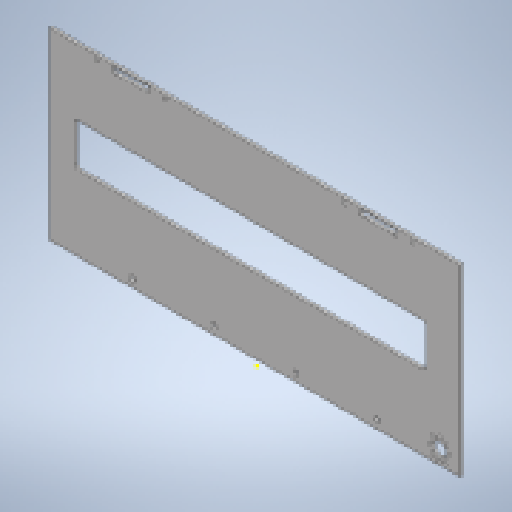
# Autodesk Inventor part: wall2
Saved by Autodesk Inventor 2024 (Build 280153000, 153)
## iProperties
Created: 2024-06-08
Part Number: wall2
Material: 一般
Document SubType Name: モデリング
Designer: right
Density: 1 g/cm^3
Appearance: 既定
Author: right
Autodesk Inventor part; units mm, degrees
ref_plane "YZ Plane" through (0, 0, 0) normal (1, 0, 0) x (0, 1, 0)
ref_plane "XZ Plane" through (0, 0, 0) normal (0, 1, 0) x (-1, 0, 0)
ref_plane "XY Plane" through (0, 0, 0) normal (0, 0, 1) x (1, 0, 0)
sketch "スケッチ1" plane through (0, 0, 0) normal (0, 0, 1) x (1, 0, 0)
  circle A0 centre (71.625, 9) radius 1.3 projected
  circle A1 centre (23.875, 9) radius 1.3 projected
  circle A2 centre (-23.875, 9) radius 1.3 projected
  circle A3 centre (-71.625, 9) radius 1.3 projected
  circle A4 centre (52.5, 109.3641) radius 0.7835 projected
  circle A5 centre (92.5, 109.3641) radius 0.7835 projected
  line L0 (62.5, 107.8641) -> (82.5, 107.8641) projected
  line L1 (82.5, 110.8641) -> (82.5, 107.8641) projected
  line L2 (62.5, 110.8641) -> (82.5, 110.8641) projected
  line L3 (62.5, 110.8641) -> (62.5, 107.8641) projected
  line L4 (-82.5, 107.8641) -> (-62.5, 107.8641) projected
  line L5 (-62.5, 110.8641) -> (-62.5, 107.8641) projected
  line L6 (-82.5, 110.8641) -> (-62.5, 110.8641) projected
  line L7 (-82.5, 110.8641) -> (-82.5, 107.8641) projected
  circle A6 centre (-92.5, 109.3641) radius 0.7835 projected
  circle A7 centre (-52.5, 109.3641) radius 0.7835 projected
  circle A8 centre (64.0053, 60.7224) radius 10 projected
  arc A9 (100, 57.7224) -> (100, 63.7224) centre (100, 60.7224) ccw projected
  circle A10 centre (100, 60.7224) radius 12.5
  arc A11 (-100, 63.7224) -> (-100, 57.7224) centre (-100, 60.7224) ccw projected
  circle A12 centre (-100, 60.7224) radius 12.5
  line L8 (100, 48.2224) -> (-100, 48.2224)
  line L9 (100, 73.2224) -> (-100, 73.2224)
  circle A13 centre (71.625, 9) radius 1.6
  circle A14 centre (23.875, 9) radius 1.6
  circle A15 centre (-23.875, 9) radius 1.6
  circle A16 centre (-71.625, 9) radius 1.6
  circle A17 centre (-92.5, 109.3641) radius 1.1
  circle A18 centre (-52.5, 109.3641) radius 1.1
  circle A19 centre (52.5, 109.3641) radius 1.1
  circle A20 centre (92.5, 109.3641) radius 1.1
  circle A21 centre (82.1, 110.4641) radius 1.1
  line L10 (82.5, 109.3641) -> (62.5, 109.3641) construction
  line L11 (82.1, 110.4641) -> (82.5, 110.8641) construction
  circle A22 centre (82.1, 108.2641) radius 1.1
  line L12 (72.5, 107.8641) -> (72.5, 109.3641) construction
  circle A23 centre (62.9, 110.4641) radius 1.1
  line L13 (62.5, 109.3641) -> (82.5, 109.3641) construction
  circle A24 centre (62.9, 108.2641) radius 1.1
  line L14 (-60.3, 107.8641) -> (60.3, 107.8641) construction
  line L15 (60.3, 110.8641) -> (-60.3, 110.8641) construction
  line L16 (0, 107.8641) -> (0, 110.8641) construction
  line L17 (-82.5, 110.8641) -> (-82.5, 107.8641)
  line L18 (-62.5, 110.8641) -> (-62.5, 107.8641)
  circle A25 centre (-82.1, 110.4641) radius 1.1
  line L19 (-82.1, 110.4641) -> (-82.5, 110.8641) construction
  circle A26 centre (-82.1, 108.2641) radius 1.1
  circle A27 centre (-62.9, 108.2641) radius 1.1
  circle A28 centre (-62.9, 110.4641) radius 1.1
  line L20 (-110, 111.8641) -> (120, 111.8641) construction
  line L21 (110, 4.5) -> (-110, 4.5) construction
  line L22 (-120, 111.8641) -> (120, 111.8641)
  line L23 (120, 111.8641) -> (120, 4.5)
  line L24 (120, 4.5) -> (-120, 4.5)
  line L25 (-120, 4.5) -> (-120, 111.8641)
  line L26 (100, 48.2224) -> (100, 73.2224)
  line L27 (100, 73.2224) -> (100, 73.2224)
  line L28 (100, 48.2224) -> (100, 48.2224)
  line L29 (-95, 48.2224) -> (-105, 48.2224)
  line L30 (-105, 48.2224) -> (-105, 73.2224)
  line L31 (-105, 73.2224) -> (-95, 73.2224)
  line L32 (-95, 73.2224) -> (-95, 48.2224)
  line L33 (-95, 48.2224) -> (-105, 73.2224) construction
  line L34 (-105, 48.2224) -> (-95, 73.2224) construction
  point P0 (0, 0)
  point P1 (-82.5, 109.3641)
  point P2 (-62.5, 109.3641)
  point P3 (-62.5, 109.3641)
  point P4 (-82.5, 109.3641)
  point P5 (62.5, 109.4394)
  point P6 (63.9247, 110.8641)
  point P7 (81.0753, 110.8641)
  point P8 (82.5, 109.4394)
  point P9 (82.5, 109.2888)
  point P10 (81.0753, 107.8641)
  point P11 (63.9247, 107.8641)
  point P12 (62.5, 109.2888)
  point P13 (-62.5, 109.4394)
  point P14 (-62.5, 109.2888)
  point P15 (-63.9247, 107.8641)
  point P16 (-81.0753, 107.8641)
  point P17 (-82.5, 109.2888)
  point P18 (-82.5, 109.4394)
  point P19 (-81.0753, 110.8641)
  point P20 (-63.9247, 110.8641)
  point P21 (-100, 73.2224)
  point P22 (-100, 48.2224)
  dimension "d0" = 3.2
  dimension "d1" = 3.2
  dimension "d2" = 3.2
  dimension "d3" = 3.2
  dimension "d4" = 2.2
  dimension "d5" = 2.2
  dimension "d6" = 2.2
  dimension "d7" = 2.2
  dimension "d8" = 2.2
  dimension "d9" = 45
  dimension "d10" = 20
  dimension "d11" = 20
  dimension "d14" = 25
  dimension "d16" = 15
  dimension "d17" = 20
  constraints: 46 end point, 18 centre point, 13 symmetric about line, 10 coincident, 8 midpoint, 7 tangent, 4 parallel, 4 point on circle, 2 horizontal, 2 horizontal alignment, 2 perpendicular, 1 equal radius, 1 point on line, 1 vertical, 7 other
  measures "d0" diameter of A13
  measures "d1" diameter of A14
  measures "d2" diameter of A15
  measures "d3" diameter of A16
  measures "d4" diameter of A17
  measures "d5" diameter of A18
  measures "d6" diameter of A19
  measures "d7" diameter of A20
  measures "d8" diameter of A21
  measures "d9" angle of L2 L11
  measures "d10" distance from line of A12.centre L25
  measures "d11" distance from line of A10.centre L23
  measures "d14" diameter of A10
  measures "d16" distance between parallel lines of L25 L30
  measures "d17" distance between parallel lines of L23 L26
extrude "押し出し1" add sketch "スケッチ1" along normal blind 1.5 contours L26 A9 | A9 L26 A10 | A12 L30 | L22 L23 L24 L25
fillet "フィレット1" radius 2 3 edges at (-105, 48.2224, 0.75) (-105, 73.2224, 0.75) (100, 73.2224, 0.75)
fillet "フィレット2" radius 2 1 edges at (100, 48.2224, 0.75)
sketch "スケッチ4" plane through (0, 0, 0) normal (0, 0, -1) x (-1, 0, 0)
  line L0 (120, 4.5) -> (-120, 4.5) projected
  line L1 (-120, 4.5) -> (-120, 111.8641) projected
  circle A0 centre (-108, 12.5) radius 4
  circle A1 centre (-108, 12.5) radius 6 construction
  circle A2 centre (-102, 12.5) radius 1.1
  circle A3 centre (-103.7574, 16.7426) radius 1.1
  circle A4 centre (-108, 18.5) radius 1.1
  circle A5 centre (-112.2426, 16.7426) radius 1.1
  circle A6 centre (-114, 12.5) radius 1.1
  circle A7 centre (-112.2426, 8.2574) radius 1.1
  circle A8 centre (-108, 6.5) radius 1.1
  circle A9 centre (-103.7574, 8.2574) radius 1.1
  line L2 (120, 4.5) -> (-120, 4.5) projected
  point P0 (0, 0)
  dimension "d27" = 12
  dimension "d26" = 8
  dimension "d28" = 2.2
  dimension "d31" = 360
  dimension "d35" = 12
  dimension "d36" = 8
  constraints: 9 centre point, 1 coincident, 1 horizontal alignment, 1 vertical alignment, 19 other
  measures "d26" diameter of A0
  measures "d28" diameter of A2
  measures "d35" distance from line of L1 A0.centre
  measures "d36" distance from line of L2 A0.centre
extrude "押し出し3" cut sketch "スケッチ4" against normal through all
sketch "スケッチ7" plane through (0, 0, 0) normal (0, 0, -1) x (-1, 0, 0)
  circle A0 centre (-108, 12.5) radius 4 projected
  circle A1 centre (-92.5444, 3.2196) radius 1.1 projected
  circle A2 centre (-108, 12.5) radius 18.0278 construction
  circle A3 centre (-93, 2.5) radius 2
  line L0 (120, 4.5) -> (-120, 4.5) construction
  circle A4 centre (-93, 2.5) radius 1.1
  circle A5 centre (-111.4615, -5.1923) radius 1.1
  circle A6 centre (-111.4615, -5.1923) radius 2
  line L1 (-91, 2.5) -> (-91, 4.5)
  line L2 (-113.1489, -6.2661) -> (-120, 4.5)
  line L3 (-93, 2.5) -> (-111.4615, -5.1923) construction
  line L4 (-98.1923, 1.9615) -> (-97.0385, -0.8077)
  line L5 (-98.1923, 1.9615) -> (-107.4231, -1.8846)
  line L6 (-107.4231, -1.8846) -> (-106.2692, -4.6538)
  line L7 (-106.2692, -4.6538) -> (-97.0385, -0.8077)
  circle A7 centre (-98.0538, -1.2308) radius 1.1
  circle A8 centre (-99.2077, 1.5385) radius 1.1
  line L8 (-101.6538, -2.7308) -> (-102.2308, -1.3462) construction
  circle A9 centre (-105.2538, -4.2308) radius 1.1
  circle A10 centre (-106.4077, -1.4615) radius 1.1
  line L9 (-97.0385, -0.8077) -> (-96.6538, -1.7308)
  line L10 (-96.6538, -1.7308) -> (-92.0542, 0.7377)
  line L11 (-106.2692, -4.6538) -> (-105.8846, -5.5769)
  line L12 (-105.8846, -5.5769) -> (-110.8762, -7.1047)
  line L13 (-91, 4.5) -> (-120, 4.5)
  point P0 (0, 0)
  point P1 (-105.3923, -1.0385)
  point P2 (-100.2231, 1.1154)
  dimension "d57" = 2.2
  dimension "d44" = 4
  dimension "d45" = 2.2
  dimension "d46" = 2.2
  dimension "d47" = 4
  dimension "d51" = 5
  dimension "d53" = 3
  dimension "d54" = 1.5
  dimension "d55" = 20
  dimension "d56" = 10
  dimension "d58" = 1
  dimension "d59" = 1
  constraints: 26 end point, 7 centre point, 7 point on circle, 5 perpendicular, 5 tangent, 3 coincident, 3 point on line, 3 symmetric about line, 2 midpoint, 2 parallel, 1 collinear, 11 other
  measures "d44" diameter of A3
  measures "d45" diameter of A4
  measures "d46" diameter of A5
  measures "d47" diameter of A6
  measures "d51" distance from line of L4 L3.start
  measures "d53" distance of L4.start L4.end
  measures "d54" distance from line of L4.start L3
  measures "d55" distance of L3.start A5.centre
  measures "d56" distance of L4.start L5.end
  measures "d58" distance of L4.end L9.end
  measures "d59" distance of L11.start L11.end
extrude "押し出し6" add sketch "スケッチ7" against normal up to surface (1.5 mm away) contours A1 A4 | A3 | L10 L9 L4 A8 L5 A10 L6 L11 L12 A6 L2 L13 A3 | A3 L13 L1 | A6 picked at (-92.1686, 3.9355)
equation "\"d11\" = d10"
equation "\"BendRadius\" = Thickness"
equation "\"BendReliefWidth\" = Thickness"
equation "\"BendReliefDepth\" = 0.5 * Thickness"
equation "\"CornerReliefSize\" = 4 * Thickness"
equation "\"MinimumRemnant\" = 2 * Thickness"
equation "\"TransitionRadius\" = BendRadius"
equation "\"JacobiRadiusSize\" = BendRadius"
equation "\"GapSize\" = Thickness"
equation "\"Thickness\" = 3.048"
